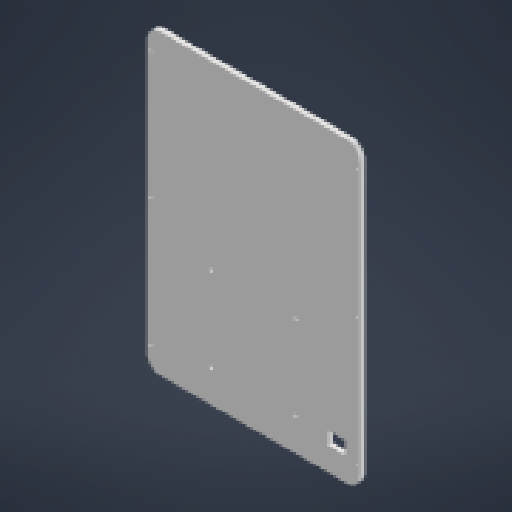
# Autodesk Inventor part: manipulation layer
Saved by Autodesk Inventor 2026.1 (Build 301233000, 233)
## iProperties
Created: 2026-03-07
Part Number: manipulation layer
Material: Generic
Document SubType Name: Modeling
Designer: momen
Density: 1 g/cm^3
Appearance: Default
Author: momen
Autodesk Inventor part; units mm, degrees
ref_plane "YZ Plane" through (0, 0, 0) normal (1, 0, 0) x (0, 1, 0)
ref_plane "XZ Plane" through (0, 0, 0) normal (0, 1, 0) x (-1, 0, 0)
ref_plane "XY Plane" through (0, 0, 0) normal (0, 0, 1) x (1, 0, 0)
sketch "Sketch1" plane through (0, 0, 0) normal (0, 0, 1) x (1, 0, 0)
  line L0 (-125, -175) -> (125, -175)
  line L1 (125, -175) -> (125, 175)
  line L2 (125, 175) -> (-125, 175)
  line L3 (-125, 175) -> (-125, -175)
  line L4 (-125, -175) -> (125, 175) construction
  line L5 (125, -175) -> (-125, 175) construction
  line L6 (-121, -150) -> (121, -150)
  line L7 (121, -150) -> (121, 150)
  line L8 (121, 150) -> (-121, 150)
  line L9 (-121, 150) -> (-121, -150)
  line L10 (-121, -150) -> (121, 150) construction
  line L11 (121, -150) -> (-121, 150) construction
  circle A0 centre (121, 150) radius 1.5
  circle A1 centre (-121, 150) radius 1.5
  circle A2 centre (-121, -150) radius 1.5
  circle A3 centre (121, -150) radius 1.5
  circle A4 centre (-121, 0) radius 1.5
  circle A5 centre (121, 0) radius 1.5
  line L12 (0, 0) -> (0, -175)
  line L13 (-125, 0) -> (125, -175)
  line L14 (125, 0) -> (-125, -175)
  circle A6 centre (49.4975, -38.0025) radius 2.05
  circle A7 centre (-49.4975, -38.0025) radius 2.05
  circle A8 centre (49.4975, -136.9975) radius 2.05
  circle A9 centre (-49.4975, -136.9975) radius 2.05
  point P0 (121, -148.5)
  point P1 (119.5, -150)
  point P2 (119.5, 150)
  point P3 (121, 148.5)
  point P4 (-121, 148.5)
  point P5 (-119.5, 150)
  point P6 (0, -87.5)
  dimension "d0" = 250
  dimension "d1" = 350
  dimension "d10" = 242
  dimension "d11" = 300
  dimension "d12" = 3
  dimension "d13" = 3
  dimension "d14" = 3
  dimension "d15" = 3
  dimension "d16" = 3
  dimension "d17" = 3
  dimension "d24" = 4.1
  dimension "d25" = 4.1
  dimension "d26" = 4.1
  dimension "d27" = 4.1
  constraints: 30 end point, 10 centre point, 10 midpoint, 4 coincident, 4 parallel, 2 horizontal, 2 perpendicular
  measures "d0" distance of L2.end L1.end
  measures "d1" distance of L1.end L0.end
  measures "d10" distance of L8.end L7.end
  measures "d11" distance of L7.end L6.end
  measures "d12" diameter of A0
  measures "d13" diameter of A1
  measures "d14" diameter of A2
  measures "d15" diameter of A3
  measures "d16" diameter of A4
  measures "d17" diameter of A5
  measures "d24" diameter of A6
  measures "d25" diameter of A7
  measures "d26" diameter of A8
  measures "d27" diameter of A9
extrude "Extrusion1" add sketch "Sketch1" along normal blind 6 contours L14 L6 L12 L0 | L3 L13 L9 A2 L6 L14 | L12 L6 L13 L0 | L3 L2 L1 L14 L7 A5 A0 L8 A1 L9 A4 L13 | L14 L12 L6 | L6 A2 L9 L13 L14 | L13 L6 A3 L7 L14 L1 | L12 L13 L6 | L9 A4 A1 L8 A0 L7 A5 L14 L13 | L14 L7 A3 L6 L13
fillet "Fillet1" radius 15 4 edges at (125, 175, 3) (125, -175, 3) (-125, -175, 3) (-125, 175, 3)
sketch "Sketch2" plane through (0, 0, 6) normal (0, 0, 1) x (1, 0, 0)
  line L0 (90, -127.5) -> (104.4, -127.5)
  line L1 (87.2, -127.5) -> (107.2, -127.5)
  line L2 (87.2, -127.5) -> (107.2, -127.5)
  line L3 (107.2, -127.5) -> (107.2, -147.5)
  line L4 (107.2, -147.5) -> (87.2, -147.5)
  line L5 (87.2, -147.5) -> (87.2, -127.5)
  line L6 (87.2, -147.5) -> (107.2, -147.5)
  line L7 (107.2, -147.5) -> (107.2, -132.5)
  line L8 (107.2, -132.5) -> (87.2, -132.5)
  line L9 (87.2, -132.5) -> (87.2, -147.5)
  point P0 (0, 0)
  point P1 (97.2, -127.5)
  dimension "d28" = 20
  dimension "d29" = 20
  dimension "d30" = 20
  dimension "d31" = 20
  dimension "d32" = 15
  constraints: 20 end point, 4 horizontal, 4 parallel, 2 midpoint, 2 perpendicular, 2 other
  measures "d28" distance of L1.start L1.end
  measures "d29" distance of L3.end L4.end
  measures "d30" distance of L2.end L3.end
  measures "d31" distance of L8.end L7.end
  measures "d32" distance of L7.end L6.end
extrude "Extrusion2" cut sketch "Sketch2" against normal through all contours L8 L3 L4 L5
body "Solid1"
